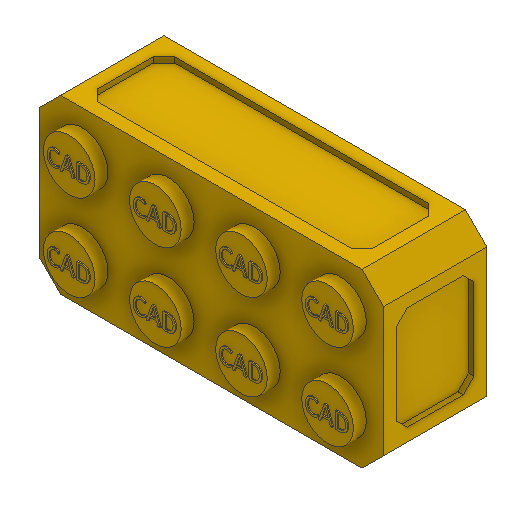
# Autodesk Inventor part: CAD 2x4 Brick
Saved by Autodesk Inventor 2026.2 (Build 302298000, 298)
## iProperties
Created: 2026-01-27
Part Number: CAD 2x4 Brick
Material: Generic
Document SubType Name: Modeling
Designer: andyeske
Density: 1 g/cm^3
Appearance: Default
Author: andyeske
Autodesk Inventor part; units mm, degrees
ref_plane "YZ Plane" through (0, 0, 0) normal (1, 0, 0) x (0, 1, 0)
ref_plane "XZ Plane" through (0, 0, 0) normal (0, 1, 0) x (-1, 0, 0)
ref_plane "XY Plane" through (0, 0, 0) normal (0, 0, 1) x (1, 0, 0)
sketch "Sketch1" plane through (0, 0, 0) normal (0, 0, 1) x (1, 0, 0)
  line L0 (-16, -8) -> (16, -8)
  line L1 (16, -8) -> (16, 8)
  line L2 (16, 8) -> (-16, 8)
  line L3 (-16, 8) -> (-16, -8)
  line L4 (-16, -8) -> (16, 8) construction
  line L5 (16, -8) -> (-16, 8) construction
  point P0 (0, 0)
  dimension "d0" = 32
  dimension "d1" = 16
  constraints: 12 end point, 2 midpoint, 2 parallel, 1 horizontal, 1 perpendicular
  measures "d0" distance of L1.end L2.end
  measures "d1" distance of L0.end L1.end
extrude "Extrusion1" add sketch "Sketch1" along normal blind 9.6
shell "Shell1" thickness 1.2 removed faces 1 at (5.3333, -2.6667, 0)
sketch "Sketch2" plane through (0, 0, 9.6) normal (0, 0, 1) x (1, 0, 0)
  circle A0 centre (-12, 4) radius 2.4
  line L0 (16, 8) -> (-16, 8) projected
  line L1 (-16, 8) -> (-16, -8) projected
  point P0 (0, 0)
  dimension "d5" = 4
  dimension "d6" = 4
  dimension "d7" = 4.8
  constraints: 1 centre point
  measures "d5" distance from line of L0 A0.centre
  measures "d6" distance from line of L1 A0.centre
  measures "d7" diameter of A0
extrude "Extrusion2" add sketch "Sketch2" along normal blind 1.2
sketch "Sketch3" plane through (-12, 4, 10.8) normal (0, 0, 1) x (1, 0, 0)
  circle A0 centre (0, 0) radius 2.4 projected
  line L0 (-2.2627, -0.8) -> (2.2627, -0.8) construction
  spline S0 degree 2 poles (-0.8586, -0.5839) (-0.8586, -0.6025) (-0.8615, -0.6311) (-0.8672, -0.6526) (-0.8758, -0.6683) (-0.9001, -0.6927) (-0.9745, -0.7399) (-1.0861, -0.7871) (-1.2306, -0.8186) (-1.3165, -0.8186) knots 0 0 0 1 2 3 4 5 6 7 8 8 8
  spline S1 degree 2 poles (-1.3165, -0.8186) (-1.4639, -0.8186) (-1.7029, -0.7199) (-1.8703, -0.5281) (-1.9605, -0.2448) (-1.9605, -0.0616) knots 0 0 0 1 2 3 4 4 4
  spline S2 degree 2 poles (-1.9605, -0.0616) (-1.9605, 0.1273) (-1.8631, 0.4221) (-1.6871, 0.6281) (-1.441, 0.7354) (-1.2922, 0.7354) knots 0 0 0 1 2 3 4 4 4
  spline S3 degree 2 poles (-1.2922, 0.7354) (-1.2264, 0.7354) (-1.1019, 0.7111) (-0.9974, 0.6739) (-0.9144, 0.6238) (-0.8829, 0.5923) (-0.8743, 0.5766) (-0.8672, 0.5537) (-0.8643, 0.5237) (-0.8643, 0.5022) knots 0 0 0 1 2 3 4 5 6 7 8 8 8
  spline S4 degree 2 poles (-0.8643, 0.5022) (-0.8643, 0.4793) (-0.8686, 0.4464) (-0.8786, 0.4235) (-0.8915, 0.4135) (-0.9015, 0.4135) knots 0 0 0 1 2 3 4 4 4
  spline S5 degree 2 poles (-0.9015, 0.4135) (-0.9173, 0.4135) (-0.9759, 0.4593) (-1.0704, 0.5136) (-1.2035, 0.5594) (-1.2965, 0.5594) knots 0 0 0 1 2 3 4 4 4
  spline S6 degree 2 poles (-1.2965, 0.5594) (-1.3981, 0.5594) (-1.5641, 0.4793) (-1.6828, 0.3219) (-1.7472, 0.0958) (-1.7472, -0.0502) knots 0 0 0 1 2 3 4 4 4
  spline S7 degree 2 poles (-1.7472, -0.0502) (-1.7472, -0.1933) (-1.6843, -0.4151) (-1.5684, -0.5639) (-1.3981, -0.6397) (-1.2907, -0.6397) knots 0 0 0 1 2 3 4 4 4
  spline S8 degree 2 poles (-1.2907, -0.6397) (-1.1992, -0.6397) (-1.0632, -0.5954) (-0.9688, -0.5396) (-0.9072, -0.4952) (-0.8886, -0.4952) knots 0 0 0 1 2 3 4 4 4
  spline S9 degree 2 poles (-0.8886, -0.4952) (-0.8815, -0.4952) (-0.8686, -0.5024) (-0.8615, -0.5224) (-0.8586, -0.5567) (-0.8586, -0.5839) knots 0 0 0 1 2 3 4 4 4
  spline S10 degree 2 poles (0.5452, -0.7285) (0.5538, -0.7542) (0.5552, -0.7857) (0.5366, -0.8029) (0.4937, -0.8072) (0.4565, -0.8072) knots 0 0 0 1 2 3 4 4 4
  spline S11 degree 2 poles (0.4565, -0.8072) (0.4207, -0.8072) (0.3778, -0.8043) (0.3549, -0.7957) (0.3449, -0.7814) (0.3391, -0.7714) knots 0 0 0 1 2 3 4 4 4
  line L1 (0.3391, -0.7714) -> (0.2104, -0.4022)
  line L2 (0.2104, -0.4022) -> (-0.4207, -0.4022)
  line L3 (-0.4207, -0.4022) -> (-0.5452, -0.7657)
  spline S12 degree 2 poles (-0.5452, -0.7657) (-0.5495, -0.7771) (-0.5609, -0.7914) (-0.5824, -0.8029) (-0.6239, -0.8072) (-0.6568, -0.8072) knots 0 0 0 1 2 3 4 4 4
  spline S13 degree 2 poles (-0.6568, -0.8072) (-0.6912, -0.8072) (-0.7341, -0.8014) (-0.7513, -0.7843) (-0.7498, -0.7528) (-0.7413, -0.727) knots 0 0 0 1 2 3 4 4 4
  line L4 (-0.7413, -0.727) -> (-0.2318, 0.6811)
  spline S14 degree 2 poles (-0.2318, 0.6811) (-0.2275, 0.6954) (-0.2118, 0.7111) (-0.1832, 0.7211) (-0.1374, 0.724) (-0.1016, 0.724) knots 0 0 0 1 2 3 4 4 4
  spline S15 degree 2 poles (-0.1016, 0.724) (-0.0644, 0.724) (-0.0157, 0.7211) (0.0157, 0.7111) (0.0315, 0.6939) (0.0358, 0.6811) knots 0 0 0 1 2 3 4 4 4
  line L5 (0.0358, 0.6811) -> (0.5452, -0.7285)
  line L6 (-0.1073, 0.5151) -> (-0.1088, 0.5151)
  line L7 (-0.1088, 0.5151) -> (-0.3706, -0.2419)
  line L8 (-0.3706, -0.2419) -> (0.1574, -0.2419)
  line L9 (0.1574, -0.2419) -> (-0.1073, 0.5151)
  spline S16 degree 2 poles (1.9647, -0.0187) (1.9647, -0.2162) (1.8646, -0.5109) (1.67, -0.7041) (1.3895, -0.8) (1.1949, -0.8) knots 0 0 0 1 2 3 4 4 4
  line L10 (1.1949, -0.8) -> (0.8729, -0.8)
  spline S17 degree 2 poles (0.8729, -0.8) (0.8471, -0.8) (0.7985, -0.7642) (0.7985, -0.7184) knots 0 0 0 1 2 2 2
  line L11 (0.7985, -0.7184) -> (0.7985, 0.6353)
  spline S18 degree 2 poles (0.7985, 0.6353) (0.7985, 0.6811) (0.8471, 0.7168) (0.8729, 0.7168) knots 0 0 0 1 2 2 2
  line L12 (0.8729, 0.7168) -> (1.2163, 0.7168)
  spline S19 degree 2 poles (1.2163, 0.7168) (1.4138, 0.7168) (1.6857, 0.6152) (1.8703, 0.4235) (1.9647, 0.1516) (1.9647, -0.0187) knots 0 0 0 1 2 3 4 4 4
  spline S20 degree 2 poles (1.753, -0.0273) (1.753, 0.0958) (1.6914, 0.3076) (1.5612, 0.4621) (1.3623, 0.5494) (1.2049, 0.5494) knots 0 0 0 1 2 3 4 4 4
  line L13 (1.2049, 0.5494) -> (1.0003, 0.5494)
  line L14 (1.0003, 0.5494) -> (1.0003, -0.6311)
  line L15 (1.0003, -0.6311) -> (1.2078, -0.6311)
  spline S21 degree 2 poles (1.2078, -0.6311) (1.3537, -0.6311) (1.5526, -0.5582) (1.6857, -0.4079) (1.753, -0.1818) (1.753, -0.0273) knots 0 0 0 1 2 3 4 4 4
  point P0 (12, -4)
  dimension "d10" = 0.8
  constraints: 2 end point, 2 horizontal, 2 point on circle
  measures "d10" distance from line of A0.centre L0
extrude "Extrusion3" add sketch "Sketch3" along normal blind 0.1 contours S0 S1 S2 S3 S4 S5 S6 S7 S8 S9 | S10 S11 L1 L2 L3 S12 S13 L4 S14 S15 L5 | S16 L10 S17 L11 S18 L12 S19
sketch "Sketch4" plane through (14.8, -6.8, 8.4) normal (0, 0, -1) x (-1, 0, 0)
  circle A0 centre (26.8, 10.8) radius 2.4 construction
  circle A1 centre (26.8, 10.8) radius 1.2
  point P0 (14.8, 6.8)
  dimension "d13" = 2.4
  constraints: 1 centre point, 1 coincident
  measures "d13" diameter of A1
extrude "Extrusion4" cut sketch "Sketch4" against normal blind 1.2
pattern_linear "Rectangular Pattern1" count 4 spacing 8 along (1, 0, 0) count 2 spacing 8 along (0, -1, 0) of "Extrusion2", "Extrusion3", "Extrusion4"
sketch "Sketch5" plane through (14.8, -6.8, 8.4) normal (0, 0, -1) x (-1, 0, 0)
  circle A0 centre (22.8, 6.8) radius 3.2
  line L0 (30.8, 14.8) -> (30.8, -1.2) projected
  line L1 (-1.2, 14.8) -> (30.8, 14.8) projected
  circle A1 centre (22.8, 6.8) radius 2.6
  point P0 (14.8, 6.8)
  dimension "d22" = 8
  dimension "d23" = 8
  dimension "d24" = 6.4
  dimension "d25" = 0.6
  constraints: 2 centre point
  measures "d22" distance from line of L0 A0.centre
  measures "d23" distance from line of L1 A0.centre
  measures "d24" diameter of A0
  measures "d25" radial gap between concentric circles of A0 A1
extrude "Extrusion5" add sketch "Sketch5" along normal up to surface (8.4 mm away)
pattern_linear "Rectangular Pattern2" count 3 spacing 8 along (1, 0, 0) of "Extrusion5"
chamfer "Chamfer1" distance 2 angle 45 4 edges at (-16, 8, 4.8) (-16, -8, 4.8) (16, -8, 4.8) (16, 8, 4.8)
sketch "Sketch6" plane through (-14, -8, 0) normal (0, -1, 0) x (1, 0, 0)
  line L0 (28, 9.6) -> (28, 0) projected
  line L1 (0, 9.6) -> (28, 9.6) projected
  line L2 (0, 0) -> (0, 9.6) projected
  line L3 (0, 0) -> (28, 0) projected
  line L4 (26.8, 8.4) -> (26.8, 1.2)
  line L5 (26.8, 1.2) -> (1.2, 1.2)
  line L6 (1.2, 1.2) -> (1.2, 8.4)
  line L7 (1.2, 8.4) -> (26.8, 8.4)
  point P0 (14, 0)
  dimension "d34" = 1.2
  constraints: 8 end point, 3 other
  measures "d34" distance between parallel lines of L1 L7
extrude "Extrusion6" cut sketch "Sketch6" against normal blind 0.5 contours L4 L5 L6 L7
sketch "Sketch7" plane through (-16, -6, 0) normal (-1, 0, 0) x (0, 0, 1)
  line L0 (9.6, 0) -> (0, 0) projected
  line L1 (9.6, 12) -> (9.6, 0) projected
  line L2 (0, 12) -> (9.6, 12) projected
  line L3 (0, 12) -> (0, 0) projected
  line L4 (8.4, 10.8) -> (8.4, 1.2)
  line L5 (8.4, 1.2) -> (1.2, 1.2)
  line L6 (1.2, 1.2) -> (1.2, 10.8)
  line L7 (1.2, 10.8) -> (8.4, 10.8)
  point P0 (0, 6)
  dimension "d37" = 1.2
  constraints: 8 end point, 3 other
  measures "d37" distance between parallel lines of L2 L7
extrude "Extrusion7" cut sketch "Sketch7" against normal blind 0.5 contours L4 L5 L6 L7
sketch "Sketch8" plane through (16, -6, 0) normal (1, 0, 0) x (0, 0, -1)
  line L0 (-1.2, 1.2) -> (-1.2, 10.8) projected
  line L1 (-8.4, 1.2) -> (-1.2, 1.2) projected
  line L2 (-8.4, 10.8) -> (-8.4, 1.2) projected
  line L3 (-1.2, 10.8) -> (-8.4, 10.8) projected
  point P0 (0, 6)
extrude "Extrusion8" cut sketch "Sketch8" against normal blind 0.5
sketch "Sketch9" plane through (-14, 8, 0) normal (0, 1, 0) x (1, 0, 0)
  line L0 (1.2, -1.2) -> (1.2, -8.4) projected
  line L1 (26.8, -1.2) -> (1.2, -1.2) projected
  line L2 (26.8, -8.4) -> (26.8, -1.2) projected
  line L3 (1.2, -8.4) -> (26.8, -8.4) projected
  point P0 (14, 0)
extrude "Extrusion9" cut sketch "Sketch9" against normal blind 0.5
chamfer "Chamfer2" distance 1 angle 45 16 edges at (12.8, -7.75, 8.4) (-12.8, -7.75, 8.4) (-12.8, -7.75, 1.2) (12.8, -7.75, 1.2) (-15.75, 4.8, 8.4) (-15.75, -4.8, 8.4) (-15.75, -4.8, 1.2) (-15.75, 4.8, 1.2) (12.8, 7.75, 1.2) (-12.8, 7.75, 1.2) (-12.8, 7.75, 8.4) (12.8, 7.75, 8.4) (15.75, 4.8, 8.4) (15.75, -4.8, 8.4) (15.75, -4.8, 1.2) (15.75, 4.8, 1.2)
chamfer "Chamfer3" distance 1.5 angle 45 4 edges at (-14.8, -6.8, 4.2) (-14.8, 6.8, 4.2) (14.8, 6.8, 4.2) (14.8, -6.8, 4.2)
body "Solid1"
